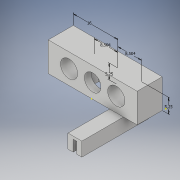
# Autodesk Inventor part: Objektträgerhalter 3a Neu
Saved by Autodesk Inventor 2018.3 (Build 223284000, 284)
## iProperties
Created: 2018-12-06
Part Number: Objektträgerhalter 3a Neu
Material: Generisch
Document SubType Name: Modeling
Designer: pgmadmin
Density: 1 g/cm^3
Appearance: Vorgabe
Author: pgmadmin
Autodesk Inventor part; units mm, degrees
ref_plane "YZ Plane" through (0, 0, 0) normal (1, 0, 0) x (0, 1, 0)
ref_plane "XZ Plane" through (0, 0, 0) normal (0, 1, 0) x (-1, 0, 0)
ref_plane "XY Plane" through (0, 0, 0) normal (0, 0, 1) x (1, 0, 0)
sketch "Skizze1" plane through (0, 0, 0) normal (0, 0, 1) x (1, 0, 0)
  point P0 (0, 0)
sketch "Skizze2" plane through (0, 0, 0) normal (0, 0, 1) x (1, 0, 0)
  line L0 (-15.5739, -1.2028) -> (16.4261, -1.2028)
  line L1 (16.4261, -1.2028) -> (16.4261, -10.2028)
  line L2 (16.4261, -10.2028) -> (-15.5739, -10.2028)
  line L3 (-15.5739, -10.2028) -> (-15.5739, -1.2028)
  point P0 (0, 0)
  dimension "d0" = 32
  dimension "d1" = 9
  constraints: 8 end point, 2 parallel, 1 horizontal, 1 perpendicular
  measures "d0" distance of L1.end L2.end
  measures "d1" distance of L0.end L1.end
extrude "Extrusion1" add sketch "Skizze2" along normal blind 10.5
sketch "Skizze3" plane through (16.4261, -10.2028, 0) normal (1, 0, 0) x (0, 0, -1)
  point P0 (0, 10.2028)
sketch "Skizze4" plane through (-15.5739, -1.2028, 0) normal (0, 1, 0) x (1, 0, 0)
  line L0 (0, 0) -> (0, -10.5) projected
  line L1 (0, 0) -> (32, 0) projected
  point P0 (15.5739, 0)
  point P1 (16, -5.25)
  point P2 (7.496, -5.25)
  point P3 (24.504, -5.25)
  dimension "d4" = 8.504
  dimension "d5" = 8.504
  dimension "d6" = 16
  dimension "d14" = 5.25
  dimension "d15" = 5.25
  measures "d4" distance of point (16, -5.25) point (7.496, -5.25)
  measures "d5" distance of point (16, -5.25) point (24.504, -5.25)
  measures "d6" distance from line of L0 point (16, -5.25)
  measures "d14" distance from line of L1 point (24.504, -5.25)
  measures "d15" vertical distance of point (15.574, 0) point (16, -5.25)
sketch "Skizze5" plane through (0, 0, 0) normal (0, 0, -1) x (-1, 0, 0)
  point P0 (0, 0)
sketch "Skizze6" plane through (0, 0, 0) normal (0, 0, -1) x (-1, 0, 0)
  line L0 (-4.8511, -7.7528) -> (3.9989, -7.7528)
  line L1 (3.9989, -7.7528) -> (3.9989, -3.6528)
  line L2 (3.9989, -3.6528) -> (-4.8511, -3.6528)
  line L3 (-4.8511, -3.6528) -> (-4.8511, -7.7528)
  line L4 (-16.4261, -10.2028) -> (15.5739, -10.2028) projected
  line L5 (15.5739, -10.2028) -> (15.5739, -1.2028) projected
  point P0 (0, 0)
  dimension "d16" = 8.85
  dimension "d17" = 4.1
  dimension "d18" = 2.45
  dimension "d19" = 11.575
  constraints: 8 end point, 2 parallel, 1 horizontal, 1 perpendicular
  measures "d16" distance of L2.end L1.end
  measures "d17" distance between parallel lines of L0 L2
  measures "d18" distance between parallel lines of L4 L0
  measures "d19" distance between parallel lines of L5 L1
extrude "Extrusion2" cut sketch "Skizze6" against normal blind 9.3
sketch "Skizze7" plane through (-15.5739, -10.2028, 0) normal (0, -1, 0) x (1, 0, 0)
  point P0 (15.5739, 0)
sketch "Skizze8" plane through (0, 0, 0) normal (0, 0, -1) x (-1, 0, 0)
  point P0 (0, 0)
sketch "Skizze9" plane through (-15.5739, -10.2028, 0) normal (0, -1, 0) x (1, 0, 0)
  line L0 (0, 0) -> (32, 0) projected
  line L1 (4.9045, 0) -> (9.9045, 0)
  line L2 (9.9045, 0) -> (9.9045, 1.2)
  line L3 (9.9045, 1.2) -> (4.9045, 1.2)
  line L4 (4.9045, 1.2) -> (4.9045, 0)
  point P0 (15.5739, 0)
  dimension "d22" = 1.2
  dimension "d23" = 5
  constraints: 8 end point, 2 parallel, 1 horizontal, 1 perpendicular, 1 point on line
  measures "d22" distance between parallel lines of L3 L0
  measures "d23" distance between parallel lines of L2 L4
extrude "Extrusion3" add sketch "Skizze9" along normal blind 15
sketch "Skizze10" plane through (0, 0, 0) normal (0, 0, -1) x (-1, 0, 0)
  line L0 (5.6694, -25.2028) -> (10.6694, -25.2028) projected
  line L1 (15.5739, -1.2028) -> (-16.4261, -1.2028) projected
  line L2 (10.6694, -25.2028) -> (5.6694, -25.2028)
  line L3 (5.6694, -25.2028) -> (5.6694, -1.2028)
  line L4 (5.6694, -1.2028) -> (10.6694, -1.2028)
  line L5 (10.6694, -1.2028) -> (10.6694, -25.2028)
  point P0 (0, 0)
  dimension "d26" = 5
  constraints: 8 end point, 2 parallel, 1 horizontal, 1 perpendicular, 1 point on line
  measures "d26" distance of L3.end L4.end
extrude "Extrusion4" add sketch "Skizze10" along normal blind 5
sketch "Skizze11" plane through (-15.5739, -25.2028, 0) normal (0, -1, 0) x (1, 0, 0)
  line L0 (4.9045, -5) -> (9.9045, -5) projected
  line L1 (6.7795, -5) -> (8.0295, -5)
  line L2 (8.0295, -5) -> (8.0295, -0.9525)
  line L3 (8.0295, -0.9525) -> (6.7795, -0.9525)
  line L4 (6.7795, -0.9525) -> (6.7795, -5)
  line L5 (9.9045, 1.2) -> (9.9045, -5) projected
  point P0 (15.5739, 0)
  dimension "d29" = 1.25
  dimension "d30" = 1.875
  dimension "d31" = 4.0475
  constraints: 8 end point, 2 parallel, 1 horizontal, 1 perpendicular, 1 point on line
  measures "d29" distance between parallel lines of L2 L4
  measures "d30" distance between parallel lines of L5 L2
  measures "d31" distance between parallel lines of L3 L0
extrude "Extrusion5" cut sketch "Skizze11" against normal blind 22
sketch "Skizze12" plane through (-15.5739, -25.2028, 0) normal (0, -1, 0) x (1, 0, 0)
  line L0 (9.9045, 1.2) -> (9.9045, 0) projected
  line L1 (4.9045, 0) -> (4.9045, 1.2) projected
  line L2 (9.9045, 1.2) -> (4.9045, 1.2)
  line L3 (4.9045, 1.2) -> (4.9045, 0)
  line L4 (4.9045, 0) -> (9.9045, 0)
  line L5 (9.9045, 0) -> (9.9045, 1.2)
  point P0 (15.5739, 0)
  constraints: 8 end point, 2 parallel, 1 horizontal, 1 perpendicular
extrude "Extrusion6" cut sketch "Skizze12" against normal blind 15
sketch "Skizze13" plane through (0, 0, 0) normal (0, 1, 0) x (-1, 0, 0)
  line L0 (5.6694, 0) -> (-16.4261, 0) projected
  line L1 (-6.5211, 0) -> (-11.5211, 0)
  line L2 (-11.5211, 0) -> (-11.5211, -5)
  line L3 (-11.5211, -5) -> (-6.5211, -5)
  line L4 (-6.5211, -5) -> (-6.5211, 0)
  line L5 (-16.4261, 0) -> (-16.4261, 10.5) projected
  point P0 (0, 0)
  dimension "d36" = 5
  dimension "d37" = 5
  dimension "d38" = 4.905
  constraints: 8 end point, 2 parallel, 1 horizontal, 1 perpendicular, 1 point on line
  measures "d36" distance of L3.end L1.start
  measures "d37" distance of L2.end L3.end
  measures "d38" distance between parallel lines of L5 L2
extrude "Extrusion7" add sketch "Skizze13" against normal blind 25.203
sketch "Skizze14" plane through (6.5211, 0, 0) normal (0, 0, 1) x (1, 0, 0)
  line L0 (5, -1.2028) -> (9.905, -1.2028) projected
  line L1 (0, 0) -> (0, -25.203) projected
  line L2 (5, -1.2028) -> (0, -1.2028)
  line L3 (0, -1.2028) -> (0, 0)
  line L4 (0, 0) -> (5, 0)
  line L5 (5, 0) -> (5, -1.2028)
  point P0 (-6.5211, 0)
  constraints: 8 end point, 2 parallel, 1 horizontal, 1 perpendicular
extrude "Extrusion8" cut sketch "Skizze14" against normal blind 25
sketch "Skizze15" plane through (0, -25.203, 0) normal (0, -1, 0) x (1, 0, 0)
  line L0 (6.5211, -5) -> (11.5211, -5) projected
  line L1 (8.3961, -5) -> (9.6461, -5)
  line L2 (9.6461, -5) -> (9.6461, -0.952)
  line L3 (9.6461, -0.952) -> (8.3961, -0.952)
  line L4 (8.3961, -0.952) -> (8.3961, -5)
  line L5 (11.5211, -5) -> (11.5211, 0) projected
  point P0 (0, 0)
  dimension "d43" = 1.25
  dimension "d44" = 4.048
  dimension "d45" = 1.875
  constraints: 8 end point, 2 parallel, 1 horizontal, 1 perpendicular, 1 point on line
  measures "d43" distance of L2.end L3.end
  measures "d44" distance of L1.end L2.end
  measures "d45" distance between parallel lines of L5 L2
extrude "Extrusion9" cut sketch "Skizze15" against normal blind 22
sketch "Skizze16" plane through (-15.5739, -25.2028, 0) normal (0, -1, 0) x (1, 0, 0)
  line L0 (0, 0) -> (4.9045, 0) projected
  line L1 (4.9045, -5) -> (9.9045, -5) projected
  line L2 (4.9045, 0) -> (9.9045, 0)
  line L3 (9.9045, 0) -> (9.9045, -5)
  line L4 (9.9045, -5) -> (4.9045, -5)
  line L5 (4.9045, -5) -> (4.9045, 0)
  point P0 (15.5739, 0)
  constraints: 8 end point, 2 parallel, 1 horizontal, 1 perpendicular
extrude "Extrusion10" cut sketch "Skizze16" against normal blind 25
hole "Bohrung2" at (0.4261, -1.2028, 5.25) direction (0, -1, 0) diameter 6 end through all
hole "Bohrung3" at (-8.0779, -1.2028, 5.25) at (8.9301, -1.2028, 5.25) direction (0, -1, 0) diameter 6.2 end through all
